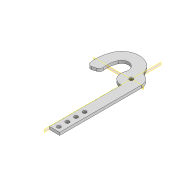
# Autodesk Inventor part: capstone hook constant radius
Saved by Autodesk Inventor 2020 (Build 240168000, 168)
## iProperties
Created: 2020-02-10
Part Number: capstone hook constant radius
Material: Generic
Document SubType Name: Modeling
Designer: ball
Density: 1 g/cm^3
Appearance: Default
Author: ball
Autodesk Inventor part; units mm, degrees
sketch "Sketch1" plane through (0, 0, 0) normal (0, 1, 0) x (-1, 0, 0)
  arc A0 (21.1036, -8.7874) -> (22.5789, 3.5742) centre (0, 0) ccw
  arc A1 (29.7917, -14.24) -> (32.529, 5.6732) centre (0, 0) ccw
  line L0 (0, 0) -> (31.7409, 9.1015) construction
  line L1 (0, 0) -> (33.02, 0) construction
  line L2 (24.8397, 7.1227) -> (28.5261, 8.1797)
  circle A2 centre (0, 0) radius 1.7
  line L3 (0, 0) -> (23.3487, -23.3487) construction
  line L4 (0, 0) -> (33.02, 0) construction
  line L5 (10.2882, -10.2882) -> (10.8225, -10.8225)
  line L6 (0, 0) -> (-10.2882, -10.2882) construction
  line L7 (0, 0) -> (25.903, 0) construction
  arc A3 (32.529, 5.6732) -> (28.5261, 8.1797) centre (29.4012, 5.1277) ccw
  arc A4 (24.8397, 7.1227) -> (22.5789, 3.5742) centre (25.7148, 4.0707) ccw
  arc A5 (8.867, -3.4788) -> (10.2882, -10.2882) centre (14.7783, -5.798) ccw
  arc A6 (10.8225, -10.8225) -> (21.1036, -8.7874) centre (15.2818, -6.3632) ccw
  arc A7 (-8.8701, -3.48) -> (-3.603, -8.8208) centre (0, 0) ccw
  arc A8 (24.6515, 7.0623) -> (24.645, 7.0668) centre (15.2818, -6.3632) ccw
  arc A9 (-0.0914, -12.3838) -> (29.7917, -14.24) centre (15.2818, -6.3632) ccw
  arc A10 (-0.0914, -12.3838) -> (-3.603, -8.8208) centre (-6.0041, -14.6994) ccw
  line L8 (-9.5283, 0) -> (-9.5243, 76.2)
  line L9 (-9.5243, 76.2) -> (0.0007, 76.2)
  line L10 (0.0007, 76.2) -> (-0.0028, 9.525)
  arc A11 (8.867, -3.4788) -> (-0.0028, 9.525) centre (0, 0) ccw
  arc A12 (-9.5283, 0) -> (-8.8701, -3.48) centre (0, 0) ccw
  circle A13 centre (-4.762, 72.2) radius 1.7
  circle A14 centre (-4.7624, 64.2) radius 1.7
  circle A15 centre (-4.7629, 56.2) radius 1.7
  circle A16 centre (-4.7633, 48.2) radius 1.7
  point P0 (21.9744, 6.3011)
  point P1 (6.7352, -6.7352)
  point P2 (-6.7352, -6.7352)
  point P3 (16.1645, -16.1645)
  point P4 (11.8424, -11.6339)
  dimension "d0" = 45.72
  dimension "d1" = 66.04
  dimension "d3" = 16
  dimension "d4" = 3.4
  dimension "d5" = 45
  dimension "d6" = 135
  dimension "d7" = 3.175
  dimension "d16" = 16.51
  dimension "d17" = 6.35
  dimension "d20" = 9.525
  dimension "d21" = 76.2
  dimension "d22" = 3.4
  dimension "d23" = 4.7625
  dimension "d24" = 4
  dimension "d27" = 8
  constraints: 28 point on circle, 22 end point, 17 centre point, 9 point on line, 9 tangent, 5 coincident, 3 horizontal, 2 equal length, 1 collinear, 1 equal radius, 1 parallel, 7 other
  measures "d0" diameter of A0
  measures "d1" diameter of A1
  measures "d3" angle of L1 L0
  measures "d4" diameter of A2
  measures "d5" angle of L3 L4
  measures "d6" angle of L6 L7
  measures "d7" radius of A3
  measures "d16" radius of A9
  measures "d17" radius of A10
  measures "d20" distance of L8.end L9.end
  measures "d21" distance of L8.start L8.end
  measures "d22" diameter of A13
  measures "d23" distance from line of L8 A13.centre
  measures "d24" distance from line of L9 A13.centre
  measures "d27" distance of A13.centre A14.centre
extrude "Extrusion1" add sketch "Sketch1" along normal mid plane 2.54
ref_plane "Work Plane1" through (0, 0.635, 0) normal (0, 1, 0) x (-1, 0, 0)
equation "\"d23\" = 0.5 * d20"
body "Solid1"
